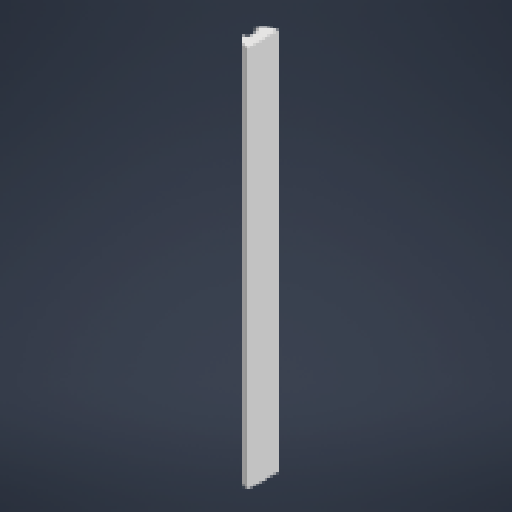
# Autodesk Inventor part: Very_long_axel
Saved by Autodesk Inventor 2026 (Build 300175050, 175E)
## iProperties
Created: 2026-06-21
Part Number: Very_long_axel
Material: Generic
Document SubType Name: Modeling
Designer: sniel
Density: 1 g/cm^3
Appearance: Default
Author: sniel
Autodesk Inventor part; units mm, degrees
ref_plane "YZ Plane" through (0, 0, 0) normal (1, 0, 0) x (0, 1, 0)
ref_plane "XZ Plane" through (0, 0, 0) normal (0, 1, 0) x (-1, 0, 0)
ref_plane "XY Plane" through (0, 0, 0) normal (0, 0, 1) x (1, 0, 0)
sketch "Sketch1" plane through (0, 0, 0) normal (0, 1, 0) x (-1, 0, 0)
  arc A0 (-3.6976, -1.5257) -> (-0.0535, -3.9996) centre (0, 0) ccw
  arc A1 (0.0535, 3.9996) -> (-3.6555, 1.624) centre (0, 0) ccw
  circle A2 centre (0, 0) radius 4
  line L0 (2.5, 1.575) -> (5.5, 1.575)
  line L1 (5.5, 1.575) -> (5.5, -1.575)
  line L2 (5.5, -1.575) -> (2.5, -1.575)
  line L3 (2.5, -1.575) -> (2.5, 1.575)
  line L4 (2.5, 1.575) -> (5.5, -1.575) construction
  line L5 (5.5, 1.575) -> (2.5, -1.575) construction
  line L6 (0, 4.5435) -> (0, -6)
  point P0 (4, 0)
  point P1 (3.6769, 1.575)
  point P2 (0.0535, 3.9996)
  point P3 (0, 4)
  point P4 (0, -4)
  point P5 (3.6769, -1.575)
  dimension "d0" = 3
  dimension "d1" = 3.15
  constraints: 14 end point, 4 point on circle, 2 centre point, 2 midpoint, 2 parallel, 1 coincident, 1 horizontal, 1 perpendicular, 4 other
  measures "d0" distance of L1.end L2.end
  measures "d1" distance of L0.end L1.end
extrude "Extrusion1" add sketch "Sketch1" along normal blind 100 contours L6 A1 A2 L0 L3 L2
body "Solid1"
